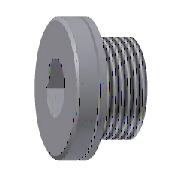
# Autodesk Inventor part: "E 2076/14"
Saved by Autodesk Inventor 2021.3 (Build 253353000, 353)
## iProperties
Created: 2020-01-21
Part Number: "E 2076/14"
Material: 2.0401
Description: Shut-off screw
Document SubType Name: Modeling
Designer: Rémi Heredero
Standard Revision: 1
Manufacturer: MEUSBURGER
Language: en-US
Size Designation: "14"
Categories: <MemberInstance><Categories><Category DisplayName="Mold" InternalName="349578f2-f4d4-4954-8c09-8e99297a61c0" Mnemonic="MOLD"><Category DisplayName="Cooling Components" InternalName="b2dbc6b9-fad2-4d9c-821a-3daa8a90842f" Mnemonic="COOLING COMPONENTS"><Category DisplayName="Pipe Plugs" InternalName="5fea04de-990e-4759-90c9-89e348c80af7" Mnemonic="PIPE PLUGS"><CategoryParameter DisplayName="Nominal Diameter" InternalName="5dc06a2d-8380-4f19-aab1-c62947a9878c" Mnemonic="NOMINAL DIAMETER"/><CategoryParameter DisplayName="Nominal Length" InternalName="961455a2-a607-461c-98e8-4545e4e151e8" Mnemonic="NOMINAL LENGTH"/><Category DisplayName="Shoulder" InternalName="10961ae6-84ca-42b3-88bd-adf826b8c2d0" Mnemonic="SHOULDER"><CategoryParameter DisplayName="Shoulder Height" InternalName="252b9f2b-a23a-492a-beeb-32b9135c699e" Mnemonic="SHOULDER HEIGHT"/><CategoryParameter DisplayName="Shoulder Diameter" InternalName="914bc0fa-d49e-4df9-8827-1b8cdc69fce1" Mnemonic="SHOULDER DIAMETER"/></Category></Category></Category></Category><Category DisplayName="DataType" InternalName="23b78d0f-2648-40c6-8793-ca6db495c9e8" Mnemonic="DATATYPE"><CategoryParameter DisplayName="DisplayName" InternalName="05415f3d-3907-474b-a020-eb9d644f4cf3" Mnemonic="DISPLAYNAME"/><CategoryParameter DisplayName="Standard" InternalName="0c0a119c-1e12-4c84-803f-101930972f5e" Mnemonic="STANDARD"/><CategoryParameter DisplayName="Description" InternalName="13903e3d-64b1-4950-80da-f627842ea37f" Mnemonic="DESCRIPTION"/><CategoryParameter DisplayName="Designation" InternalName="2675968c-4ce5-49e0-a4f5-552d29089031" Mnemonic="DESIGNATION"/><CategoryParameter DisplayName="Default Row" InternalName="2af9ec52-faaa-4026-b378-f9fa4afca842" Mnemonic="DEFAULTROW"/><CategoryParameter DisplayName="Folder Name" InternalName="3f06958e-8713-4116-9be7-ed6184ecc97b" Mnemonic="FOLDERNAME"/><CategoryParameter DisplayName="Revision Guid" InternalName="45a75005-10b1-4dfc-8d6d-dfe629f0b93c" Mnemonic="REVISIONGUID"/><CategoryParameter DisplayName="FileName" InternalName="8b46a4cc-9585-4fed-90c3-899f57e09a73" Mnemonic="FILENAME"/><CategoryParameter DisplayName="StdsOrg" InternalName="8f5914e1-4693-403f-8ab5-d37768198c9d" Mnemonic="STDSORG"/><CategoryParameter DisplayName="Family Version" InternalName="914462f6-6e19-4b14-ba84-155b9680b1d0" Mnemonic="FAMILYREVISION"/><CategoryParameter DisplayName="Standard Revision" InternalName="91d5a463-65c2-4fde-b823-3b7fea5e8e17" Mnemonic="STANDARDREVISION"/><CategoryParameter DisplayName="Member Revision" InternalName="a65d44b9-392f-4f4f-857b-e4b3d54996fe" Mnemonic="MEMBERREVISION"/><CategoryParameter DisplayName="ClipFormat" InternalName="bc51e27b-3422-4e78-93ef-cec197ddf230" Mnemonic="CLIPFORMAT"/><CategoryParameter DisplayName="Manufacturer" InternalName="cd6c7a72-a28a-4e50-99a9-2c7f4e13e5ad" Mnemonic="MANUFACTURER"/><CategoryParameter DisplayName="InternalName" InternalName="cf1d0246-76d9-4b4a-8305-fa0409afb5c1" Mnemonic="INTERNALNAME"/><CategoryParameter DisplayName="IsMetric" InternalName="e2385c5b-1ea4-4823-96a8-8de651266ec3" Mnemonic="ISMETRIC"/><Category DisplayName="Part" InternalName="c0e0b642-3bcb-4cc8-9e80-f96d35c4afa4" Mnemonic="PART"><CategoryParameter DisplayName="Part Number" InternalName="016b6077-bfbe-49bd-92c9-d8d59c39c941" Mnemonic="PARTNUMBER"/><CategoryParameter DisplayName="Stock Number" InternalName="4dba7c1c-e26c-444e-836c-b08b433409a8" Mnemonic="STOCKNUMBER"/><CategoryParameter DisplayName="Material Key" InternalName="5c9a8adb-dd2b-4535-b97f-0a94a95fe41f" Mnemonic="MATERIALKEY"/><CategoryParameter DisplayName="Material" InternalName="818a152a-d3c3-49ca-80ee-df7d91421b8e" Mnemonic="MATERIAL"/></Category></Category></Categories><FamilyTemplate Id="E 2076"><FamilyTemplateParameters><FamilyTemplateParameter ObjectType="kUserParameterObject" ValueType="xs:double" Id="1" ObjectReferenceKey="d1_"/><FamilyTemplateParameter ObjectType="kUserParameterObject" ValueType="xs:double" Id="2" ObjectReferenceKey="SW"/><FamilyTemplateParameter ObjectType="kUserParameterObject" ValueType="xs:double" Id="3" ObjectReferenceKey="l3"/><FamilyTemplateParameter ObjectType="kUserParameterObject" ValueType="xs:double" Id="4" ObjectReferenceKey="s_"/><FamilyTemplateParameter ObjectType="kUserParameterObject" ValueType="xs:double" Id="5" ObjectReferenceKey="l_"/><FamilyTemplateParameter ObjectType="kUserParameterObject" ValueType="xs:double" Id="6" ObjectReferenceKey="d3"/><FamilyTemplateParameter ObjectType="kUserParameterObject" ValueType="xs:double" Id="7" ObjectReferenceKey="l1"/><FamilyTemplateParameter ObjectType="kThreadFeatureObject" ValueType="xs:string" Id="8" ObjectReferenceKey="10020000100000007a2d0000000000008000000000000000" SubObjectId="ThreadInfo"><FamilyTemplateParameter ObjectType="" ValueType="xs:string" Id="9" SubObjectId="ThreadType"/><FamilyTemplateParameter ObjectType="" ValueType="xs:string" Id="10" SubObjectId="ThreadDesignation"/><FamilyTemplateParameter ObjectType="" ValueType="xs:string" Id="11" SubObjectId="ThreadDirection"/><FamilyTemplateParameter ObjectType="" ValueType="xs:string" Id="12" SubObjectId="ThreadClass"/></FamilyTemplateParameter><FamilyTemplateParameter ObjectType="kPartComponentDefinitionObject" ValueType="xs:string" Id="13" SubObjectId="Material"/><FamilyTemplateParameter ObjectType="kPropertyObject" ValueType="xs:string" Id="22" ObjectReferenceKey="{32853F0F-3444-11d1-9E93-0060B03C1CA6}" SubObjectId="5"/><FamilyTemplateParameter ObjectType="kPropertyObject" ValueType="xs:string" Id="23" ObjectReferenceKey="{32853F0F-3444-11d1-9E93-0060B03C1CA6}" SubObjectId="52"/></FamilyTemplateParameters></FamilyTemplate><CategoryParameterMap><ParamToTemplateMap><ParamToTemplate CategoryParameter="//CategoryParameter[@InternalName='2af9ec52-faaa-4026-b378-f9fa4afca842']" ConstantValue="1"/><ParamToTemplate CategoryParameter="//CategoryParameter[@InternalName='bc51e27b-3422-4e78-93ef-cec197ddf230']" ConstantValue="CF_INVENTOR.STDPARTS"/><ParamToTemplate CategoryParameter="//CategoryParameter[@InternalName='e2385c5b-1ea4-4823-96a8-8de651266ec3']" ConstantValue="true"/><ParamToTemplate CategoryParameter="//CategoryParameter[@InternalName='cf1d0246-76d9-4b4a-8305-fa0409afb5c1']" ConstantValue="cb925001-fba6-4b41-ba76-a5780d948e86"/><ParamToTemplate CategoryParameter="//CategoryParameter[@InternalName='45a75005-10b1-4dfc-8d6d-dfe629f0b93c']" ConstantValue="020a5fe4-0e0d-4582-8238-aa667f07a47c"/><ParamToTemplate CategoryParameter="//CategoryParameter[@InternalName='3f06958e-8713-4116-9be7-ed6184ecc97b']" ConstantValue="E 2076"/><ParamToTemplate CategoryParameter="//CategoryParameter[@InternalName='8f5914e1-4693-403f-8ab5-d37768198c9d']" TemplateParameter="17"/><ParamToTemplate CategoryParameter="//CategoryParameter[@InternalName='0c0a119c-1e12-4c84-803f-101930972f5e']" TemplateParameter="18"/><ParamToTemplate CategoryParameter="//CategoryParameter[@InternalName='91d5a463-65c2-4fde-b823-3b7fea5e8e17']" ConstantValue="1"/><ParamToTemplate CategoryParameter="//CategoryParameter[@InternalName='cd6c7a72-a28a-4e50-99a9-2c7f4e13e5ad']" ConstantValue="MEUSBURGER"/><ParamToTemplate CategoryParameter="//CategoryParameter[@InternalName='13903e3d-64b1-4950-80da-f627842ea37f']" ConstantValue="Shut-off screw"/><ParamToTemplate CategoryParameter="//CategoryParameter[@InternalName='05415f3d-3907-474b-a020-eb9d644f4cf3']" ConstantValue="E 2076"/><ParamToTemplate CategoryParameter="//CategoryParameter[@InternalName='914462f6-6e19-4b14-ba84-155b9680b1d0']" ConstantValue="1"/><ParamToTemplate CategoryParameter="//CategoryParameter[@InternalName='bc51e27b-3422-4e78-93ef-cec197ddf230']" ConstantValue="CF_INVENTOR.STDPARTS"/><ParamToTemplate CategoryParameter="//CategoryParameter[@InternalName='8b46a4cc-9585-4fed-90c3-899f57e09a73']" ConstantValue="&quot;E 2076-14&quot;"/><ParamToTemplate CategoryParameter="//CategoryParameter[@InternalName='a65d44b9-392f-4f4f-857b-e4b3d54996fe']" ConstantValue="CC3BEE47-4DE4-4F69-9785-B07D3C4E39E7"/><ParamToTemplate CategoryParameter="//CategoryParameter[@InternalName='2675968c-4ce5-49e0-a4f5-552d29089031']" TemplateParameter="23"/><ParamToTemplate CategoryParameter="//CategoryParameter[@InternalName='818a152a-d3c3-49ca-80ee-df7d91421b8e']" TemplateParameter="13"/><ParamToTemplate CategoryParameter="//CategoryParameter[@InternalName='016b6077-bfbe-49bd-92c9-d8d59c39c941']" TemplateParameter="22"/><ParamToTemplate CategoryParameter="//CategoryParameter[@InternalName='5dc06a2d-8380-4f19-aab1-c62947a9878c']" TemplateParameter="1"/><ParamToTemplate CategoryParameter="//CategoryParameter[@InternalName='914bc0fa-d49e-4df9-8827-1b8cdc69fce1']" TemplateParameter="6"/><ParamToTemplate CategoryParameter="//CategoryParameter[@InternalName='252b9f2b-a23a-492a-beeb-32b9135c699e']" TemplateParameter="3"/><ParamToTemplate CategoryParameter="//CategoryParameter[@InternalName='961455a2-a607-461c-98e8-4545e4e151e8']" TemplateParameter="5"/></ParamToTemplateMap></CategoryParameterMap></MemberInstance>
Density: 8.5 g/cm^3
Appearance: Aluminum - Dark
IsCustomPart: 0
Author: Rémi Heredero
Autodesk Inventor part; units mm, degrees
ref_plane "YZ Plane" through (0, 0, 0) normal (1, 0, 0) x (0, 1, 0)
ref_plane "XZ Plane" through (0, 0, 0) normal (0, 1, 0) x (-1, 0, 0)
ref_plane "XY Plane" through (0, 0, 0) normal (0, 0, 1) x (1, 0, 0)
sketch "Sketch1" plane through (0, 0, 0) normal (0, 1, 0) x (-1, 0, 0)
  line L0 (0, -15) -> (0, 6) projected
  line L1 (3.4641, 3) -> (9.5, 3)
  line L2 (9.5, 3) -> (9.5, 0)
  line L3 (9.5, 0) -> (7, 0)
  line L4 (7, 0) -> (7, -12)
  line L5 (7, -12) -> (0, -12)
  line L6 (0, -12) -> (0, -2.8026)
  line L7 (3.4641, 3) -> (3, 2.7321)
  line L8 (3, 2.7321) -> (3, -1)
  line L9 (0, -2.8026) -> (3, -1)
  point P0 (0, 0)
  dimension "d0" = 19
  dimension "d10" = 14
  dimension "d5" = 3
  dimension "d6" = 15
  dimension "d66" = 60
  dimension "d67" = 6
  dimension "d68" = 6.9282
  dimension "d74" = 59
  dimension "d75" = 4
  constraints: 18 end point, 2 parallel, 2 perpendicular, 2 point on line, 1 horizontal
  measures "d0" diameter of L2 L0
  measures "d10" diameter of L4 L0
  measures "d5" distance between parallel lines of L3 L1
  measures "d6" distance between parallel lines of L5 L1
  measures "d66" angle of L7 L8
  measures "d67" diameter of L8 L0
  measures "d68" diameter of L1.start L0
  measures "d74" angle of L0 L9
  measures "d75" distance from line of L1 L8.end
revolve "Revolution1" add sketch "Sketch1" angle 360 about axis through (0, 0, -10) along (0, 0, 1)
sketch "Sketch2" plane through (0, 0, 0) normal (0, 1, 0) x (-1, 0, 0)
  line L0 (7, -12) -> (7, 0) construction
  line L1 (0, -14.4) -> (0, 2.4) construction
  line L2 (7, 0) -> (5.8, -2.4)
  line L3 (5.8, -2.4) -> (7, -2.4)
  line L4 (7, 0) -> (7, -2.4)
  point P0 (0, 0)
  dimension "d72" = 2.4
  dimension "d73" = 1.2
  constraints: 6 end point, 2 perpendicular, 1 point on line
  measures "d72" distance from line of L3 L0.end
  measures "d73" distance of L2.end L3.end
revolve "Revolution2" cut sketch "Sketch2" angle 360 about axis through (0, 0, -10) along (0, 0, 1)
sketch "Sketch3" plane through (0, 0, 3) normal (0, 0, 1) x (1, 0, 0)
  line L0 (3.4641, 0) -> (1.7321, -3)
  line L1 (1.7321, -3) -> (-1.7321, -3)
  line L2 (-1.7321, -3) -> (-3.4641, 0)
  line L3 (-3.4641, 0) -> (-1.7321, 3)
  line L4 (-1.7321, 3) -> (1.7321, 3)
  line L5 (1.7321, 3) -> (3.4641, 0)
  point P0 (0, 0)
  point P1 (0, 0)
  dimension "d69" = 6
  constraints: 12 end point, 1 coincident, 1 horizontal alignment, 13 other
  measures "d69" distance between parallel lines of L2 L5
extrude "Extrusion1" cut sketch "Sketch3" against normal up to surface round surface about axis through (0, 0, -1.9013) along (0, 0, 1) radius 1.5 half angle 59 far side no
sketch "Sketch4" plane through (0, 0, 0) normal (1, 0, 0) x (0, 1, 0)
  line L0 (7, 0) -> (5.8, -2.4) projected
  line L1 (0, -3.48) -> (0, 4.08) projected
  line L2 (6.65, -0.7) -> (9.5, -0.7)
  line L3 (9.5, -0.7) -> (9.5, -1.7)
  line L4 (9.5, -1.7) -> (6.15, -1.7)
  line L5 (9.5, 0) -> (9.5, 3) projected
  point P0 (6.4, -1.2)
  point P1 (9.5, -1.2)
  dimension "d77" = 1
  constraints: 6 end point, 2 horizontal, 2 midpoint, 2 point on line, 1 collinear, 1 horizontal alignment
  measures "d77" distance between parallel lines of L4 L2
revolve "Revolution3" add sketch "Sketch4" angle 360 about axis through (0, 0, -10) along (0, 0, 1)
thread "Thread1" size "M14x1.5" class "6g" standard "ISO Metric profile" full length
chamfer "Chamfer1" distance 0.4642 angle 45 2 edges at (9.5, 0, 3) (7, 0, -12)
equation "\"d0\" = d3"
equation "\"d10\" = d1_"
equation "\"d5\" = l3"
equation "\"d6\" = l_"
equation "\"d66\" = d100"
equation "\"d67\" = SW"
equation "\"d68\" = 1.1547 * SW"
equation "\"d72\" = 0.2 * l1"
equation "\"d73\" = 0.1 * l1"
equation "\"d77\" = s_"
equation "\"d69\" = SW"
equation "\"d70\" = 0.6 * SW"
equation "\"d60\" = 0.07737 * SW"
equation "\"SW\" = 6"
equation "\"l3\" = 3"
equation "\"l1\" = 12"
equation "\"l_\" = 15"
equation "\"d3\" = 19"
equation "\"d1_\" = 14"
equation "\"d100\" = 60deg"
equation "\"s_\" = 1"
body "Solid1"
